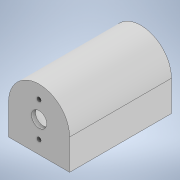
# Autodesk Inventor part: bancada
Saved by Autodesk Inventor 2021 (Build 250183000, 183)
## iProperties
Created: 2022-10-24
Part Number: bancada
Material: Generic
Document SubType Name: Modeling
Designer: felip
Density: 1 g/cm^3
Appearance: Default
Author: felip
Autodesk Inventor part; units mm, degrees
ref_plane "YZ Plane" through (0, 0, 0) normal (1, 0, 0) x (0, 1, 0)
ref_plane "XZ Plane" through (0, 0, 0) normal (0, 1, 0) x (-1, 0, 0)
ref_plane "XY Plane" through (0, 0, 0) normal (0, 0, 1) x (1, 0, 0)
sketch "Sketch1" plane through (0, 0, 0) normal (0, 0, 1) x (1, 0, 0)
  circle A0 centre (0, 15) radius 12.5
  arc A1 (15, 15) -> (-15, 15) centre (0, 15) ccw
  line L0 (-15, 15) -> (-15, 0)
  line L1 (15, 15) -> (15, 0)
  line L2 (15, 0) -> (-15, 0)
  point P0 (0, 0)
  dimension "d0" = 25
  dimension "d1" = 30
  dimension "d2" = 15
  constraints: 6 end point, 2 centre point, 2 point on circle, 2 tangent, 2 vertical, 1 coincident, 1 perpendicular
  measures "d0" diameter of A0
  measures "d1" diameter of A1
  measures "d2" distance of point (0, 0) A0.centre
extrude "Extrusion1" add sketch "Sketch1" along normal blind 50
sketch "Sketch2" plane through (0, 0, 50) normal (0, 0, 1) x (1, 0, 0)
  circle A0 centre (0, 15) radius 12.5 construction
  line L0 (0, 27.5) -> (0, 2.5) construction
  circle A1 centre (0, 15) radius 12.5
  point P0 (0, 0)
  constraints: 2 end point, 2 point on circle, 1 centre point, 1 coincident, 1 concentric, 1 vertical
extrude "Extrusion2" add sketch "Sketch2" against normal blind 2
sketch "Sketch3" plane through (0, 0, 50) normal (0, 0, 1) x (1, 0, 0)
  circle A0 centre (0, 15) radius 12.5 construction
  line L0 (0, 2.5) -> (0, 27.5) construction
  circle A1 centre (0, 23.5) radius 1
  circle A2 centre (0, 6.5) radius 1
  circle A3 centre (0, 15) radius 3.75
  point P0 (0, 0)
  dimension "d7" = 2
  dimension "d8" = 2
  dimension "d9" = 8.5
  dimension "d10" = 17
  dimension "d11" = 7.5
  constraints: 3 centre point, 2 end point, 2 point on circle, 2 point on line, 1 coincident, 1 vertical
  measures "d7" diameter of A1
  measures "d8" diameter of A2
  measures "d9" distance of A0.centre A1.centre
  measures "d10" distance of A1.centre A2.centre
  measures "d11" diameter of A3
extrude "Extrusion3" cut sketch "Sketch3" against normal blind 2.5
thread "Thread1" size "M2x0.4" class "6H" standard "ANSI Metric M Profile" full length
thread "Thread2" size "M2x0.4" class "6H" standard "ANSI Metric M Profile" full length
body "Solid1"
